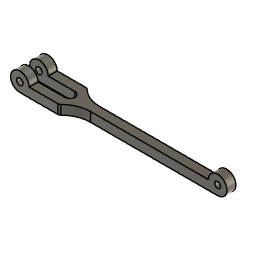
bar (Autodesk Fusion 360 design; units mm, degrees)
Autodesk Fusion 360 part; units mm, degrees
note: some values were not read from the file. Chosen so that the rebuilt part matches the saved one: that a step has no effect; which face or edge a step refers to. Set by a fixed rule: which sketch regions a step uses.
sketch "mainBody" plane through (0, 0, 0) normal (0, 0, 1) x (1, 0, 0)
  line L0 (0, 0) -> (50, 0)
  line L1 (50, 0) -> (50, -1.5)
  line L2 (50, -1.5) -> (0, -1.5)
  line L3 (0, -1.5) -> (0, 0)
  line L4 (0, 0) -> (50, 0)
  line L5 (50, 0) -> (50, 1.5)
  line L6 (50, 1.5) -> (0, 1.5)
  line L7 (0, 1.5) -> (0, 0)
  line L8 (0, 0) -> (-1.1, 0)
  line L9 (-1.1, 0) -> (-1.1, 4.7)
  line L10 (-1.1, 4.7) -> (0, 4.7)
  line L11 (0, 4.7) -> (0, 0)
  line L12 (0, 0) -> (-1.1, 0)
  line L13 (-1.1, 0) -> (-1.1, -4.7)
  line L14 (-1.1, -4.7) -> (0, -4.7)
  line L15 (0, -4.7) -> (0, 0)
  line L16 (-1.1, -4.7) -> (-13.2, -4.7)
  line L17 (-13.2, -4.7) -> (-13.2, -1.7)
  line L18 (-13.2, -1.7) -> (-1.1, -1.7)
  line L19 (-1.1, -1.7) -> (-1.1, -4.7)
  line L20 (-1.1, 4.7) -> (-13.2, 4.7)
  line L21 (-13.2, 4.7) -> (-13.2, 1.7)
  line L22 (-13.2, 1.7) -> (-1.1, 1.7)
  line L23 (-1.1, 1.7) -> (-1.1, 4.7)
  line L24 (50, -1.5) -> (46.25, -1.5)
  line L25 (46.25, -1.5) -> (39.25, -1.5)
  line L26 (39.25, -1.5) -> (39.25, -0.5)
  line L27 (39.25, -0.5) -> (46.25, -0.5)
  line L28 (46.25, -0.5) -> (46.25, -1.5)
  dimension "d10" = 1.5
  dimension "d11" = 50
  dimension "d12" = 50
  dimension "d13" = 1.5
  dimension "d14" = 4.7
  dimension "d15" = 4.7
  dimension "d16" = 1.1
  dimension "d17" = 1.1
  dimension "d18" = 3
  dimension "d19" = 12.1
  dimension "d20" = 12.1
  dimension "d21" = 3
  dimension "d25" = 3.75
  dimension "d26" = 1
  dimension "d27" = 7
  dimension "d68" = 3.4
  constraint horizontal L0
  constraint vertical L1
  constraint horizontal L2
  constraint vertical L3
  constraint coincident L0.start L3.end
  constraint horizontal L4
  constraint vertical L5
  constraint horizontal L6
  constraint vertical L7
  constraint horizontal L8
  constraint vertical L9
  constraint horizontal L10
  constraint vertical L11
  constraint horizontal L12
  constraint vertical L13
  constraint horizontal L14
  constraint vertical L15
  constraint horizontal L16
  constraint vertical L17
  constraint horizontal L18
  constraint vertical L19
  constraint horizontal L20
  constraint vertical L21
  constraint horizontal L22
  constraint vertical L23
  constraint perpendicular L1 L24
  constraint horizontal L25
  constraint vertical L26
  constraint horizontal L27
  constraint vertical L28
  measures "d10" distance of L0.start L2.end
  measures "d11" distance of L1.end L2.end
  measures "d12" distance of L5.end L6.end
  measures "d13" distance of L0.start L6.end
  measures "d14" distance of L0.start L10.end
  measures "d15" distance of L0.start L14.end
  measures "d16" distance of L9.end L10.end
  measures "d17" distance of L13.end L14.end
  measures "d18" distance of L13.end L18.end
  measures "d19" distance of L13.end L16.end
  measures "d20" distance of L9.end L20.end
  measures "d21" distance of L20.end L21.end
  measures "d25" distance of L1.end L24.end
  measures "d26" distance of L24.end L27.end
  measures "d27" distance of L24.end L25.end
  measures "d68" distance of L18.end L22.end
extrude "Extrude1" add sketch "mainBody" along normal blind 3.125 contours L0 L4 L5 L6 L7 L11 | L0 L1 L2 L3 L4 L15 L24 L26 L27 L28 | L7 L8 L9 L10 L11 L12 L23 | L3 L8 L12 L13 L14 L15 L19 | L9 L20 L21 L22 L23 | L13 L16 L17 L18 L19
sketch "backHole" plane through (0, -1.5, 0) normal (0, -1, 0) x (1, 0, 0)
  line L0 (0, 0) -> (39.25, 0)
  line L1 (39.25, 0) -> (39.25, 3.125)
  line L2 (39.25, 3.125) -> (0, 3.125)
  line L3 (0, 3.125) -> (0, 0)
  circle A0 centre (50, 3.125) radius 3.125
  circle A1 centre (50, 3.125) radius 1
  line L4 (0, 0) -> (50, 0)
  line L5 (50, 0) -> (50, 3.125)
  line L6 (50, 3.125) -> (0, 3.125)
  line L7 (0, 3.125) -> (0, 0)
  dimension "d30" = 6.25
  dimension "d31" = 2
  dimension "d65" = 50
  dimension "d66" = 3.125
  constraint concentric A0 A1
  constraint horizontal L4
  constraint vertical L5
  constraint horizontal L6
  constraint vertical L7
  constraint coincident A0.centre A1.centre
  constraint coincident L0.start L3.end
  measures "d30" diameter of A0
  measures "d31" diameter of A1
  measures "d65" distance of L0.start L4.end
  measures "d66" distance of L0.start L2.end
extrude "Extrude2" cut sketch "backHole" against normal blind 3 contours A1 L5 L6 | A1 L5 L6
extrude "Extrude3" add sketch "backHole" against normal blind 3 contours A0 A1 L5 L6 | A0 A1 L5 L6
sketch "oneFrontHole" plane through (0, -1.7, 0) normal (0, 1, 0) x (-1, 0, 0)
  line L0 (1.1, 0) -> (13.2, 0)
  line L1 (13.2, 0) -> (13.2, 3.125)
  line L2 (13.2, 3.125) -> (1.1, 3.125)
  line L3 (1.1, 3.125) -> (1.1, 0)
  circle A0 centre (13.2, 3.125) radius 3.125
  circle A1 centre (13.2, 3.125) radius 1.1
  dimension "d40" = 6.25
  dimension "d41" = 2.2
  constraint coincident L1.end L2.start
  constraint concentric A0 A1
  measures "d40" diameter of A0
  measures "d41" diameter of A1
extrude "Extrude4" cut sketch "oneFrontHole" against normal blind 3 contours L1 L2 A1 picked at (12.4704, 3.0728)
extrude "Extrude5" add sketch "oneFrontHole" against normal blind 3 contours L1 L2 A0 A1 picked at (12.4537, 5.4515)
sketch "twoFrontHole" plane through (0, 1.7, 0) normal (0, -1, 0) x (1, 0, 0)
  line L0 (-13.2, 0) -> (-1.1, 0)
  line L1 (-1.1, 0) -> (-1.1, 3.125)
  line L2 (-1.1, 3.125) -> (-13.2, 3.125)
  line L3 (-13.2, 3.125) -> (-13.2, 0)
  circle A0 centre (-13.2, 3.125) radius 3.125
  circle A1 centre (-13.2, 3.125) radius 1.1
  dimension "d46" = 6.25
  dimension "d47" = 2.2
  constraint coincident L2.end L3.start
  measures "d46" diameter of A0
  measures "d47" diameter of A1
extrude "Extrude6" cut sketch "twoFrontHole" against normal blind 3 contours L2 L3 A1 picked at (-12.4704, 3.0728)
extrude "Extrude7" add sketch "twoFrontHole" against normal blind 3 contours L2 L3 A0 A1 picked at (-14.7245, 1.2154)
extrude "Extrude8" add sketch "mainBody" along normal blind 3.125 contours L2 L25 L26 L27 L28
fillet "Fillet1" radius 10 1 edges at (0, -1.5, 1.5625)
fillet "Fillet2" radius 10 1 edges at (0, 1.5, 1.5625)
fillet "Fillet3" radius 1 2 edges at (0, 4.7, 1.5625) (0, -4.7, 1.5625)
fillet "Fillet4" [no effect]
fillet "Fillet5" [no effect]
sketch "Sketch7" plane through (0, 0, 3.125) normal (0, 0, 1) x (-1, 0, 0)
  line L0 (10.075, -4.7) -> (10.075, -1.7)
  line L1 (10.075, -1.7) -> (1.1, -1.7)
  line L2 (1.1, -1.7) -> (1.1, 1.7)
  line L3 (1.1, 1.7) -> (10.075, 1.7)
  line L4 (10.075, 1.7) -> (10.075, 4.7)
  line L5 (-46.875, 1.5) -> (-46.875, -1.5)
  circle A0 centre (1.1, 0) radius 1.7
  arc A1 (0.4242, 4.7) -> (-0.281, 4.4091) centre (0.4242, 3.7) ccw
  arc A2 (-7.3321, 1.5) -> (-0.281, 4.4091) centre (-7.3321, 11.5) ccw
  line L6 (-7.3321, 1.5) -> (-46.875, 1.5)
  line L7 (-46.875, -1.5) -> (-7.3321, -1.5)
  arc A3 (-0.281, -4.4091) -> (-7.3321, -1.5) centre (-7.3321, -11.5) ccw
  arc A4 (-0.281, -4.4091) -> (0.4242, -4.7) centre (0.4242, -3.7) ccw
  line L8 (0.4242, -4.7) -> (10.075, -4.7)
  line L9 (10.075, 4.7) -> (0.4242, 4.7)
  dimension "d69" = 3.4
  constraint midpoint L2 A0.centre
  measures "d69" diameter of A0
extrude "Extrude9" cut sketch "Sketch7" against normal blind 3.125 contours L2 A0 | L2 A0
fillet "Fillet6" [no effect]
equation "mainBarLength = 50 mm"
equation "mainBarWidth = 3 mm"
equation "mainBarHeight = 3.125 mm"
equation "tBarLength = 9.4 mm"
equation "tBarWidth = 4.4 mm"
equation "hBarHeight = 8.8 mm" comment "6.8mm"
equation "hBarWidth = 3 mm"
equation "outerCircle = 6.25 mm"
equation "innerCircle = 2.2 mm"
equation "d10 = mainBarWidth / 2"
equation "d11 = mainBarLength"
equation "d12 = mainBarLength"
equation "d13 = mainBarWidth / 2"
equation "d14 = tBarLength / 2"
equation "d15 = tBarLength / 2"
equation "d16 = tBarWidth / 4"
equation "d17 = tBarWidth / 4"
equation "d18 = hBarWidth"
equation "d19 = hBarHeight + tBarWidth * 3 / 4"
equation "d20 = hBarHeight + tBarWidth * 3 / 4"
equation "d21 = hBarWidth"
equation "insertDist = 3.75 mm"
equation "insertWidth = 7 mm"
equation "insertHeight = 1 mm"
equation "d25 = insertDist"
equation "d26 = insertHeight"
equation "d27 = insertWidth"
equation "d28 = mainBarHeight"
equation "d30 = outerCircle"
equation "d31 = innerCircleSmallDiam"
equation "d34 = -mainBarWidth"
equation "d36 = -mainBarWidth"
equation "d40 = outerCircle"
equation "d41 = innerCircle"
equation "d42 = -hBarWidth"
equation "d44 = -hBarWidth"
equation "d46 = outerCircle"
equation "d47 = innerCircle"
equation "d48 = -hBarWidth"
equation "d50 = -hBarWidth"
equation "d52 = mainBarHeight"
equation "pointerFingerOffset = 25 mm"
equation "d65 = mainBarLength"
equation "d66 = mainBarHeight"
equation "innerCircleSmallDiam = 2 mm"
equation "d70 = -mainBarHeight"
